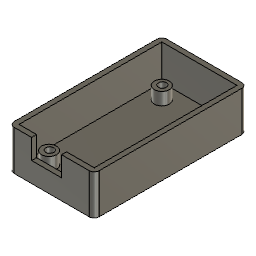
enclosure (Autodesk Fusion 360 design; units mm, degrees)
part number: 2026-07-02-23-05-05-164
Autodesk Fusion 360 part; units mm, degrees
note: some values were not read from the file. Set by a fixed rule: which sketch regions a step uses.
sketch "草图1" plane through (0, 0, 0) normal (0, 0, 1) x (1, 0, 0)
  line L0 (17, -30.5) -> (-17, -30.5)
  line L1 (-17, -30.5) -> (-17, 30.5)
  line L2 (-17, 30.5) -> (17, 30.5)
  line L3 (17, 30.5) -> (17, -30.5)
  line L4 (17, -30.5) -> (-17, 30.5) construction
  line L5 (-17, -30.5) -> (17, 30.5) construction
  dimension "d1" = 34
  dimension "d2" = 61
  constraint horizontal L0
  constraint perpendicular L0 L1
  constraint parallel L0 L2
  constraint parallel L1 L3
  constraint coincident L4 origin
  constraint coincident L5 origin
  measures "d1" distance of L1.end L2.end
  measures "d2" distance of L0.end L1.end
extrude "拉伸1" add sketch "草图1" along normal blind 16
shell "抽壳1" thickness 2 removed faces 1 at (5.6667, -10.1667, 16)
sketch "草图2" plane through (0, 0, 2) normal (0, 0, 1) x (-1, 0, 0)
  line L0 (-15, -28.5) -> (15, -28.5)
  line L1 (15, -28.5) -> (15, 28.5)
  line L2 (15, 28.5) -> (-15, 28.5)
  line L3 (-15, 28.5) -> (-15, -28.5)
  circle A0 centre (12.3837, -25.5684) radius 3
  dimension "d6" = 6
  measures "d6" diameter of A0
extrude "拉伸2" add sketch "草图2" along normal blind 5 contours L0 L1 A0 picked at (12.7417, -24.831)
delete_face "删除面1" 1 faces at (-11.6033, 28.4651, 5.3333)
sketch "草图3" plane through (0, 0, 2) normal (0, 0, 1) x (-1, 0, 0)
  line L0 (15, -28.5) -> (15, 28.5)
  line L1 (15, 28.5) -> (-15, 28.5)
  line L2 (-15, 28.5) -> (-15, -28.5)
  line L3 (-15, -28.5) -> (15, -28.5)
  circle A0 centre (9, -22.5) radius 3
  dimension "d12" = 6
  dimension "d13" = 6
  dimension "d14" = 6
  measures "d12" diameter of A0
  measures "d13" distance of L0 A0.centre
  measures "d14" distance of L3 A0.centre
extrude "拉伸3" add sketch "草图3" along normal blind 5 contours A0
pattern_linear "R-阵列1" count 2 spacing 18 along (1, 0, 0) count 2 spacing 45 along (0, -1, 0) of "拉伸3"
hole "孔1" at (-8.9823, 22.7476, 7) direction (0, 0, -1) diameter 3.2 depth 5 tip angle 180
pattern_linear "R-阵列2" count 2 spacing 18 along (1, 0, 0) count 2 spacing 45 along (0, -1, 0) of "孔1"
sketch "草图4" plane through (0, -30.5, 0) normal (0, -1, 0) x (1, 0, 0)
  line L0 (-17, 0) -> (17, 0)
  line L1 (17, 0) -> (17, 16)
  line L2 (17, 16) -> (-17, 16)
  line L3 (-17, 16) -> (-17, 0)
  line L4 (-8, 16) -> (4, 16)
  line L5 (4, 16) -> (4, 8)
  line L6 (4, 8) -> (-8, 8)
  line L7 (-8, 8) -> (-8, 16)
  dimension "d28" = 12
  dimension "d29" = 8
  dimension "d30" = 9
  dimension "d31" = 8
  constraint horizontal L4
  constraint vertical L5
  constraint horizontal L6
  constraint vertical L7
  measures "d28" distance of L4.start L4.end
  measures "d29" distance of L4.start L6.end
  measures "d30" distance of L3 L7
  measures "d31" distance of L0 L6
extrude "拉伸4" cut sketch "草图4" along normal blind 20 and the other way blind 20 contours L2 L4 L5 L6 L7
fillet "圆角1" radius 2 4 edges at (17, -30.5, 8) (-17, -30.5, 8) (17, 30.5, 8) (-17, 30.5, 8)
